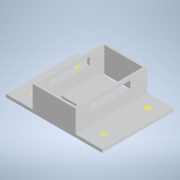
# Autodesk Inventor part: voltometer_socket
Saved by Autodesk Inventor 2021 (Build 250183000, 183)
## iProperties
Created: 2021-03-03
Part Number: voltometer_socket
Material: Generic
Document SubType Name: Modeling
Designer: Mateusz
Density: 1 g/cm^3
Appearance: Default
Author: Mateusz
Autodesk Inventor part; units mm, degrees
ref_plane "YZ Plane" through (0, 0, 0) normal (1, 0, 0) x (0, 1, 0)
ref_plane "XZ Plane" through (0, 0, 0) normal (0, 1, 0) x (-1, 0, 0)
sketch "Sketch1" plane through (0, 0, 0) normal (0, 1, 0) x (-1, 0, 0)
  line L0 (0, 0) -> (26, 0)
  line L1 (26, 0) -> (26, -45.5)
  line L2 (26, -45.5) -> (0, -45.5)
  line L3 (0, -45.5) -> (0, 0)
  line L4 (-1.5, 0) -> (-1.5, -45.5)
  line L5 (-1.5, -45.5) -> (-1.5, -47)
  line L6 (-1.5, -47) -> (26, -47)
  line L7 (26, -47) -> (27.5, -47)
  line L8 (27.5, -47) -> (27.5, 0)
  line L9 (27.5, 0) -> (27.5, 1.5)
  line L10 (27.5, 1.5) -> (-1.5, 1.5)
  line L11 (-1.5, 1.5) -> (-1.5, 0)
  dimension "d0" = 26
  dimension "d1" = 45.5
  dimension "d3" = 1.5
  dimension "d4" = 1.5
  dimension "d5" = 1.5
  constraints: 24 end point, 7 point on line, 5 perpendicular, 2 parallel, 1 horizontal
  measures "d0" distance of L0.start L0.end
  measures "d1" distance of L0.end L1.end
  measures "d3" distance of L4.end L5.end
  measures "d4" distance of L6.end L7.end
  measures "d5" distance of L8.end L9.end
extrude "Extrusion1" add sketch "Sketch1" along normal blind 15
sketch "Sketch2" plane through (1.5, 0, 1.5) normal (1, 0, 0) x (0, 0, -1)
  line L0 (9.5, 13) -> (37, 13)
  line L1 (37, 13) -> (37, 8)
  line L2 (9.5, 13) -> (9.5, 8)
  line L3 (37, 8) -> (9.5, 8)
  point P0 (1.5, 0)
  point P1 (48.5, 0)
  constraints: 8 end point, 1 horizontal, 1 perpendicular
extrude "Extrusion2" cut sketch "Sketch2" against normal up to surface (29 mm away)
sketch "Sketch3" plane through (0, 0, 0) normal (0, -1, 0) x (1, 0, 0)
  line L0 (1.5, 1.5) -> (1.5, -47) projected
  line L1 (-27.5, 1.5) -> (1.5, 1.5) projected
  line L2 (-27.5, -47) -> (-27.5, 1.5) projected
  line L3 (1.5, -47) -> (-27.5, -47) projected
  line L4 (0, 0) -> (-26, 0) projected
  line L5 (0, -45.5) -> (0, 0) projected
  line L6 (-26, -45.5) -> (0, -45.5) projected
  line L7 (-26, 0) -> (-26, -45.5) projected
  line L8 (0, 0) -> (-26, 0) projected
  line L9 (-26, 0) -> (-26, -3)
  line L10 (-26, 0) -> (-26, -45.5) projected
  line L11 (-26, -3) -> (0, -3)
  line L12 (0, -45.5) -> (0, 0) projected
  line L13 (-26, -45.5) -> (-26, -42.5)
  line L14 (-26, -42.5) -> (0, -42.5)
  line L15 (0, -42.5) -> (-26, -42.5)
  line L16 (-26, -42.5) -> (-26, -3)
  line L17 (-26, -3) -> (0, -3)
  line L18 (0, -3) -> (0, -42.5)
  dimension "d15" = 3
  dimension "d16" = 3
  constraints: 16 end point, 4 point on line, 3 perpendicular, 2 parallel, 1 horizontal
  measures "d15" distance of L4.end L9.end
  measures "d16" distance of L6.start L13.end
extrude "Extrusion3" add sketch "Sketch3" along normal blind 2 contours L0 L3 L2 L1 | L5 L14 L7 L11
sketch "Sketch5" plane through (0, -2, 0) normal (0, -1, 0) x (1, 0, 0)
  line L0 (0, -3) -> (-26, -3) projected
  line L1 (0, -35.5) -> (0, -8) projected
  line L2 (-26, -3) -> (0, -3)
  line L3 (0, -3) -> (0, -16.2813)
  line L4 (0, -16.2813) -> (-26, -16.2813)
  line L5 (-26, -16.2813) -> (-26, -3)
  point P0 (0, 0)
  point P1 (0, -8)
  constraints: 8 end point, 2 parallel, 1 horizontal, 1 perpendicular, 1 point on line
ref_plane "Work Plane1" through (-23.6, 15, -43.3) normal (0, 1, 0) x (0, 0, 1)
extrude "Extrusion4" cut sketch "Sketch5" against normal up to surface (17 mm away)
sketch "Sketch6" plane through (1.5, 15, 1.5) normal (1, 0, 0) x (0, 0, -1)
  line L0 (0, -17) -> (48.5, -17) projected
  line L1 (0, -17) -> (0, -15)
  line L2 (0, 0) -> (0, -17) projected
  line L3 (0, -15) -> (48.5, -15)
  line L4 (48.5, -17) -> (48.5, 0) projected
  line L5 (48.5, -17) -> (48.5, -15)
  line L6 (48.5, -17) -> (0, -17)
  point P0 (1.5, -15)
  dimension "d21" = 2
  constraints: 8 end point, 2 perpendicular, 2 point on line, 1 collinear
  measures "d21" distance of L0.start L1.end
extrude "Extrusion5" add sketch "Sketch6" along normal blind 18
sketch "Sketch7" plane through (-27.5, 15, -47) normal (-1, 0, 0) x (0, 0, 1)
  line L0 (0, -15) -> (48.5, -15) projected
  line L1 (48.5, -15) -> (48.5, -17) projected
  line L2 (48.5, -17) -> (0, -17) projected
  line L3 (0, -17) -> (0, -15) projected
  point P0 (47, -15)
extrude "Extrusion6" add sketch "Sketch7" along normal blind 18
sketch "Sketch8" plane through (1.5, 0, 1.5) normal (0, 1, 0) x (1, 0, 0)
  circle A0 centre (9, 9.8591) radius 1.4501 projected
  circle A1 centre (9.0001, 39.8592) radius 1.4502 projected
  circle A2 centre (-38, 9.859) radius 1.4499 projected
  circle A3 centre (-38, 39.8587) radius 1.4497 projected
  line L0 (9, 9.8591) -> (9, 19.7911)
  circle A4 centre (9, 19.7911) radius 4.767
  line L1 (-38, 9.859) -> (-38, 19.7911)
  circle A5 centre (-38, 19.7911) radius 4.767
  point P0 (-1.5, 1.5)
  dimension "d26" = 9.932
  dimension "d27" = 9.534
  constraints: 4 end point, 2 centre point, 2 coincident, 2 vertical
  measures "d26" distance of L0.start L0.end
  measures "d27" diameter of A4
extrude "Extrusion7" cut sketch "Sketch8" against normal up to surface (2 mm away)
body "Solid1"
